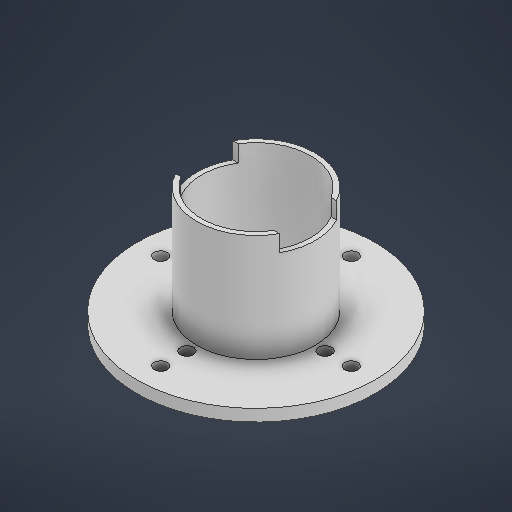
# Autodesk Inventor part: holder
Saved by Autodesk Inventor 2025 (Build 290162000, 162)
## iProperties
Created: 2024-10-04
Part Number: holder
Material: Generic
Document SubType Name: Modeling
Designer: mayhe
Density: 1 g/cm^3
Appearance: Default
Author: mayhe
Autodesk Inventor part; units mm, degrees
ref_plane "YZ Plane" through (0, 0, 0) normal (1, 0, 0) x (0, 1, 0)
ref_plane "XZ Plane" through (0, 0, 0) normal (0, 1, 0) x (-1, 0, 0)
ref_plane "XY Plane" through (0, 0, 0) normal (0, 0, 1) x (1, 0, 0)
sketch "Sketch1" plane through (0, 0, 0) normal (0, 1, 0) x (-1, 0, 0)
  circle A0 centre (0, 0) radius 50
  circle A1 centre (0, 0) radius 40
  circle A2 centre (0, -40) radius 2.75
  circle A3 centre (40, 0) radius 2.75
  circle A4 centre (0, 40) radius 2.75
  circle A5 centre (-40, 0) radius 2.75
  circle A6 centre (0, 0) radius 22.9
  circle A7 centre (0, 0) radius 24.9
  line L0 (31.0901, 12) -> (-31.0901, 12)
  line L1 (-31.0901, 12) -> (-31.0901, -12)
  line L2 (-31.0901, -12) -> (31.0901, -12)
  line L3 (31.0901, -12) -> (31.0901, 12)
  line L4 (31.0901, 12) -> (-31.0901, -12) construction
  line L5 (-31.0901, 12) -> (31.0901, -12) construction
  point P0 (-21.8177, 12)
  point P1 (-19.5041, 12)
  point P2 (19.5041, 12)
  point P3 (21.8177, 12)
  point P4 (21.8177, -12)
  point P5 (19.5041, -12)
  point P6 (-19.5041, -12)
  point P7 (-21.8177, -12)
  dimension "d1" = 80
  dimension "d0" = 100
  dimension "d2" = 5.5
  dimension "d5" = 360
  dimension "d7" = 45.8
  dimension "d8" = 2
  dimension "d9" = 24
  constraints: 12 end point, 7 centre point, 3 coincident, 2 midpoint, 2 parallel, 1 horizontal, 1 perpendicular, 1 vertical alignment, 11 other
  measures "d0" diameter of A0
  measures "d2" diameter of A2
  measures "d7" diameter of A6
  measures "d8" radial gap between concentric circles of A6 A7
  measures "d9" distance of L1.end L0.end
extrude "Extrusion1" add sketch "Sketch1" along normal blind 5 contours A0 | A3 A1 A2 A5 A4 | A6 L2 L0 | A6 L0 A7 L2 | L0 A6 | A6 L0 A7 | L2 A7 A6 | A6 L2 | A6 L2 A7 L0 | L0 L3 L2 A7 | A7 L2 L1 L0
extrude "Extrusion2" add sketch "Sketch1" along normal blind 50.1 contours A6 L0 A7 | L2 A7 A6
extrude "Extrusion3" add sketch "Sketch1" along normal blind 43.1 contours A6 L0 A7 L2 | A6 L2 A7 L0
sketch "Sketch2" plane through (0, 5, 0) normal (0, 1, 0) x (1, 0, 0)
  circle A0 centre (0, 0) radius 29
  circle A1 centre (29, 0) radius 2.75
  circle A2 centre (0, 29) radius 2.75
  circle A3 centre (-29, 0) radius 2.75
  circle A4 centre (0, -29) radius 2.75
  dimension "d16" = 58
  dimension "d17" = 5.5
  dimension "d20" = 360
  constraints: 4 centre point, 1 coincident, 1 horizontal alignment, 11 other
  measures "d17" diameter of A1
extrude "Extrusion4" cut sketch "Sketch2" against normal blind 43.1 contours A0 A1 | A0 A1 | A2 A0 | A0 A2 | A4 A0 | A0 A4 | A3 A0 | A0 A3
body "Solid1"
